Autodesk Fusion 360 part; units mm, degrees
note: some values were not read from the file. Set by a fixed rule: which sketch regions a step uses.
(part 15 of 15)
  line L12343 (-11.7716, -39.6941) -> (-12.0521, -39.6609)
  line L12344 (1.5382, -40.9023) -> (1.397, -40.7821)
  line L12345 (12.7412, -42.5744) -> (12.5951, -42.6886)
  line L12346 (11.5659, -41.0915) -> (11.7302, -41.0056)
  line L12347 (11.908, -40.9533) -> (12.0927, -40.9365)
  line L12348 (1.1512, -39.9247) -> (1.2072, -39.7479)
  line L12349 (1.397, -40.7821) -> (1.2819, -40.6368)
  line L12350 (11.2028, -42.2362) -> (11.1517, -42.0579)
  line L12351 (1.2072, -39.7479) -> (1.2966, -39.5855)
  line L12352 (1.2819, -40.6368) -> (1.1971, -40.4719)
  line L12353 (12.0662, -42.8362) -> (11.8821, -42.8143)
  line L12354 (2.424, -41.0079) -> (2.2454, -41.0578)
  line L12355 (1.5602, -39.3273) -> (1.7245, -39.2414)
  line L12356 (1.1971, -40.4719) -> (1.146, -40.2937)
  line L12357 (1.2966, -39.5855) -> (1.4157, -39.4434)
  line L12358 (-9.9098, -38.6322) -> (-10.0593, -38.8719)
  line L12359 (-9.7568, -37.1383) -> (-9.6973, -37.4145)
  line L12360 (-9.7956, -38.3738) -> (-9.9098, -38.6322)
  line L12361 (-12.8274, -39.3326) -> (-13.0464, -39.1543)
  line L12362 (1.146, -40.2937) -> (1.1305, -40.1089)
  line L12363 (-13.5251, -38.4617) -> (-13.6145, -38.1937)
  line L12364 (-13.6653, -37.9158) -> (-13.6764, -37.6335)
  line L12365 (1.7245, -39.2414) -> (1.9024, -39.189)
  line L12366 (11.7057, -42.757) -> (11.5439, -42.6665)
  line L12367 (-11.0893, -35.7847) -> (-10.8258, -35.8867)
  line L12368 (11.3022, -41.3497) -> (11.4214, -41.2077)
  line L12369 (11.8821, -42.8143) -> (11.7057, -42.757)
  line L12370 (1.8764, -41.05) -> (1.7001, -40.9927)
  line L12371 (2.7355, -40.8102) -> (2.5894, -40.9243)
  line L12372 (-11.3645, -35.7209) -> (-11.0893, -35.7847)
  line L12373 (2.9483, -40.5086) -> (2.8567, -40.6698)
  line L12374 (-10.8258, -35.8867) -> (-10.5793, -36.0247)
  line L12375 (1.7001, -40.9927) -> (1.5382, -40.9023)
  line L12376 (2.5894, -40.9243) -> (2.424, -41.0079)
  line L12377 (-10.1565, -36.3974) -> (-9.9887, -36.6247)
  line L12378 (3.0068, -40.3327) -> (2.9483, -40.5086)
  line L12379 (2.0605, -41.072) -> (1.8764, -41.05)
  line L12380 (-6.1433, -37.7909) -> (-6.0004, -37.9091)
  line L12381 (-16.025, -37.5022) -> (-16.1711, -37.6163)
  line L12382 (-9.6973, -37.4145) -> (-9.6774, -37.6963)
  line L12383 (-16.1711, -37.6163) -> (-16.3366, -37.6999)
  line L12384 (-7.6089, -38.7499) -> (-7.6244, -38.5652)
  line L12385 (-9.7189, -38.1019) -> (-9.7956, -38.3738)
  line L12386 (-7.4731, -39.0931) -> (-7.5578, -38.9282)
  line L12387 (-10.6864, -39.4336) -> (-10.9411, -39.5559)
  line L12388 (-5.7249, -38.605) -> (-5.7481, -38.7889)
  line L12389 (-5.8067, -38.9649) -> (-5.8982, -39.1261)
  line L12390 (-15.7538, -37.0247) -> (-15.8123, -37.2006)
  line L12391 (-7.4584, -38.0417) -> (-7.3392, -37.8997)
  line L12392 (-17.0605, -37.6847) -> (-17.2224, -37.5943)
  line L12393 (-17.2224, -37.5943) -> (-17.3635, -37.4741)
  line L12394 (-17.3635, -37.4741) -> (-17.4787, -37.3288)
  line L12395 (-17.4787, -37.3288) -> (-17.5635, -37.1639)
  line L12396 (-12.4716, -35.8608) -> (-12.2051, -35.7672)
  line L12397 (-10.4515, -39.2766) -> (-10.6864, -39.4336)
  line L12398 (-7.6038, -38.3809) -> (-7.5477, -38.2042)
  line L12399 (-13.4734, -36.8164) -> (-13.3315, -36.5722)
  line L12400 (-16.7001, -37.764) -> (-16.8842, -37.742)
  line L12401 (-9.6813, -37.8219) -> (-9.7189, -38.1019)
  line L12402 (-7.5477, -38.2042) -> (-7.4584, -38.0417)
  line L12403 (-5.7245, -38.5785) -> (-5.7249, -38.605)
  line L12404 (-17.5635, -37.1639) -> (-17.6146, -36.9857)
  line L12405 (-10.9411, -39.5559) -> (-11.2105, -39.6411)
  line L12406 (-13.0464, -39.1543) -> (-13.2382, -38.9468)
  line L12407 (-6.3064, -37.7027) -> (-6.1433, -37.7909)
  line L12408 (-5.7962, -38.2164) -> (-5.7426, -38.3939)
  line L12409 (-5.7426, -38.3939) -> (-5.7245, -38.5785)
  line L12410 (-7.3579, -39.2384) -> (-7.4731, -39.0931)
  line L12411 (-7.5578, -38.9282) -> (-7.6089, -38.7499)
  line L12412 (-15.8019, -36.4522) -> (-15.7483, -36.6297)
  line L12413 (-6.6679, -37.6285) -> (-6.4835, -37.6479)
  line L12414 (-15.8123, -37.2006) -> (-15.9039, -37.3618)
  line L12415 (-16.8842, -37.742) -> (-17.0605, -37.6847)
  line L12416 (-6.331, -39.4642) -> (-6.5096, -39.514)
  line L12417 (-5.8982, -39.1261) -> (-6.0194, -39.2664)
  line L12418 (-6.0004, -37.9091) -> (-5.8833, -38.0527)
  line L12419 (-11.928, -35.7121) -> (-11.6459, -35.6966)
  line L12420 (-6.6944, -39.5282) -> (-6.8785, -39.5063)
  line L12421 (-6.4835, -37.6479) -> (-6.3064, -37.7027)
  line L12422 (-11.6459, -35.6966) -> (-11.3645, -35.7209)
  line L12423 (-7.0549, -39.449) -> (-7.2167, -39.3585)
  line L12424 (-16.312, -35.9384) -> (-16.1489, -36.0266)
  line L12425 (-6.1655, -39.3806) -> (-6.331, -39.4642)
  line L12426 (-7.2167, -39.3585) -> (-7.3579, -39.2384)
  line L12427 (-11.4891, -39.6874) -> (-11.7716, -39.6941)
  line L12428 (-5.8833, -38.0527) -> (-5.7962, -38.2164)
  line L12429 (-6.5096, -39.514) -> (-6.6944, -39.5282)
  line L12430 (-12.9522, -36.1553) -> (-12.7223, -35.991)
  line L12431 (-12.2051, -35.7672) -> (-11.928, -35.7121)
  line L12432 (-16.5152, -37.7498) -> (-16.7001, -37.764)
  line L12433 (-12.7223, -35.991) -> (-12.4716, -35.8608)
  line L12434 (-16.1489, -36.0266) -> (-16.0061, -36.1448)
  line L12435 (-16.0061, -36.1448) -> (-15.8889, -36.2885)
  line L12436 (-15.9039, -37.3618) -> (-16.025, -37.5022)
  line L12437 (-15.7305, -36.8407) -> (-15.7538, -37.0247)
  line L12438 (-6.0194, -39.2664) -> (-6.1655, -39.3806)
  line L12439 (-13.6476, -37.3525) -> (-13.5795, -37.0783)
  line L12440 (-6.8785, -39.5063) -> (-7.0549, -39.449)
  line L12441 (-15.7483, -36.6297) -> (-15.7302, -36.8142)
  line L12442 (-5.7481, -38.7889) -> (-5.8067, -38.9649)
  line L12443 (-7.6244, -38.5652) -> (-7.6038, -38.3809)
  line L12444 (-17.464, -36.2775) -> (-17.3449, -36.1354)
  line L12445 (-16.3366, -37.6999) -> (-16.5152, -37.7498)
  line L12446 (-29.447, -36.1256) -> (-29.7017, -36.2479)
  line L12447 (-28.4379, -34.3883) -> (-28.4419, -34.5139)
  line L12448 (-30.4065, -32.3886) -> (-30.1251, -32.4129)
  line L12449 (-32.1594, -35.4064) -> (-32.2857, -35.1537)
  line L12450 (-24.9039, -34.4829) -> (-24.761, -34.6011)
  line L12451 (-31.2322, -32.5528) -> (-30.9657, -32.4592)
  line L12452 (-24.6438, -34.7447) -> (-24.5568, -34.9084)
  line L12453 (-31.0858, -36.2805) -> (-31.3459, -36.1703)
  line L12454 (-6.8525, -37.6453) -> (-6.6679, -37.6285)
  line L12455 (-31.7128, -32.8473) -> (-31.4829, -32.683)
  line L12456 (-25.2441, -34.3399) -> (-25.067, -34.3947)
  line L12457 (-24.5672, -35.6569) -> (-24.6588, -35.8181)
  line L12458 (-32.3401, -33.7703) -> (-32.234, -33.5084)
  line L12459 (-24.5087, -35.4809) -> (-24.5672, -35.6569)
  line L12460 (-31.9988, -35.6388) -> (-32.1594, -35.4064)
  line L12461 (-17.0361, -35.9334) -> (-16.8582, -35.881)
  line L12462 (-28.4579, -34.1065) -> (-28.4379, -34.3883)
  line L12463 (-28.7493, -33.3167) -> (-28.6151, -33.5653)
  line L12464 (-24.5568, -34.9084) -> (-24.5032, -35.0859)
  line L12465 (-32.234, -33.5084) -> (-32.0921, -33.2642)
  line L12466 (-24.4855, -35.297) -> (-24.5087, -35.4809)
  line L12467 (-31.807, -35.8463) -> (-31.9988, -35.6388)
  line L12468 (-29.7017, -36.2479) -> (-29.971, -36.3331)
  line L12469 (-29.2121, -35.9686) -> (-29.447, -36.1256)
  line L12470 (-29.971, -36.3331) -> (-30.2497, -36.3794)
  line L12471 (-32.4259, -34.6078) -> (-32.437, -34.3255)
  line L12472 (-28.9171, -33.0894) -> (-28.7493, -33.3167)
  line L12473 (-29.1153, -32.8881) -> (-28.9171, -33.0894)
  line L12474 (-28.5174, -33.8303) -> (-28.4579, -34.1065)
  line L12475 (-30.8127, -36.3529) -> (-31.0858, -36.2805)
  line L12476 (-7.3392, -37.8997) -> (-7.1947, -37.7835)
  line L12477 (-17.3449, -36.1354) -> (-17.2004, -36.0193)
  line L12478 (-30.5322, -36.3861) -> (-30.8127, -36.3529)
  line L12479 (-16.8582, -35.881) -> (-16.6735, -35.8642)
  line L12480 (-16.4892, -35.8836) -> (-16.312, -35.9384)
  line L12481 (-29.3399, -32.7167) -> (-29.1153, -32.8881)
  line L12482 (-30.2497, -36.3794) -> (-30.5322, -36.3861)
  line L12483 (-17.6301, -36.8009) -> (-17.6094, -36.6167)
  line L12484 (-28.4419, -34.5139) -> (-28.4795, -34.7939)
  line L12485 (-29.5864, -32.5787) -> (-29.3399, -32.7167)
  line L12486 (-15.7302, -36.8142) -> (-15.7305, -36.8407)
  line L12487 (-24.5032, -35.0859) -> (-24.4851, -35.2705)
  line L12488 (-31.3459, -36.1703) -> (-31.588, -36.0246)
  line L12489 (-15.8889, -36.2885) -> (-15.8019, -36.4522)
  line L12490 (-24.4851, -35.2705) -> (-24.4855, -35.297)
  line L12491 (-32.2857, -35.1537) -> (-32.3751, -34.8857)
  line L12492 (-28.6151, -33.5653) -> (-28.5174, -33.8303)
  line L12493 (-32.437, -34.3255) -> (-32.4082, -34.0445)
  line L12494 (-28.4795, -34.7939) -> (-28.5562, -35.0658)
  line L12495 (-17.5534, -36.4399) -> (-17.464, -36.2775)
  line L12496 (-30.1251, -32.4129) -> (-29.8499, -32.4767)
  line L12497 (-29.0017, -35.7802) -> (-29.2121, -35.9686)
  line L12498 (-16.6735, -35.8642) -> (-16.4892, -35.8836)
  line L12499 (-17.6094, -36.6167) -> (-17.5534, -36.4399)
  line L12500 (-17.2004, -36.0193) -> (-17.0361, -35.9334)
  line L12501 (-28.5562, -35.0658) -> (-28.6704, -35.3242)
  line L12502 (-28.6704, -35.3242) -> (-28.8199, -35.5639)
  line L12503 (-28.8199, -35.5639) -> (-29.0017, -35.7802)
  line L12504 (-29.8499, -32.4767) -> (-29.5864, -32.5787)
  line L12505 (-17.6146, -36.9857) -> (-17.6301, -36.8009)
  line L12506 (-7.1947, -37.7835) -> (-7.0304, -37.6976)
  line L12507 (-7.0304, -37.6976) -> (-6.8525, -37.6453)
  line L12508 (-26.3695, -35.442) -> (-26.385, -35.2572)
  line L12509 (-25.9553, -34.4755) -> (-25.791, -34.3896)
  line L12510 (-26.385, -35.2572) -> (-26.3644, -35.0729)
  line L12511 (-24.6588, -35.8181) -> (-24.78, -35.9584)
  line L12512 (-25.455, -36.2203) -> (-25.6391, -36.1983)
  line L12513 (-24.761, -34.6011) -> (-24.6438, -34.7447)
  line L12514 (-25.6391, -36.1983) -> (-25.8154, -36.141)
  line L12515 (-35.0726, -32.6304) -> (-34.9095, -32.7186)
  line L12516 (-36.2393, -34.0208) -> (-36.3241, -33.8559)
  line L12517 (-35.6448, -34.434) -> (-35.8211, -34.3767)
  line L12518 (-26.3083, -34.8962) -> (-26.219, -34.7337)
  line L12519 (-36.3241, -33.8559) -> (-36.3752, -33.6777)
  line L12520 (-36.1054, -32.8274) -> (-35.9609, -32.7113)
  line L12521 (-25.067, -34.3947) -> (-24.9039, -34.4829)
  line L12522 (-30.6886, -32.4041) -> (-30.4065, -32.3886)
  line L12523 (-48.347, -29.2707) -> (-48.1005, -29.4087)
  line L12524 (-47.6777, -29.7814) -> (-47.5099, -30.0087)
  line L12525 (-48.1005, -29.4087) -> (-47.8759, -29.5801)
  line L12526 (-34.5624, -33.1442) -> (-34.5089, -33.3217)
  line L12527 (-35.6188, -32.573) -> (-35.4341, -32.5562)
  line L12528 (-35.0972, -34.3919) -> (-35.2758, -34.4418)
  line L12529 (-47.5099, -30.0087) -> (-47.3757, -30.2573)
  line L12530 (-35.2758, -34.4418) -> (-35.4607, -34.456)
  line L12531 (-34.4908, -33.5062) -> (-34.4911, -33.5327)
  line L12532 (-31.9172, -33.0423) -> (-31.7128, -32.8473)
  line L12533 (-24.9261, -36.0726) -> (-25.0916, -36.1562)
  line L12534 (-25.4285, -34.3205) -> (-25.2441, -34.3399)
  line L12535 (-25.8154, -36.141) -> (-25.9773, -36.0506)
  line L12536 (-25.9773, -36.0506) -> (-26.1185, -35.9304)
  line L12537 (-26.3184, -35.6202) -> (-26.3695, -35.442)
  line L12538 (-34.9095, -32.7186) -> (-34.7667, -32.8368)
  line L12539 (-47.3757, -30.2573) -> (-47.2779, -30.5223)
  line L12540 (-34.7667, -32.8368) -> (-34.6495, -32.9805)
  line L12541 (-47.8759, -29.5801) -> (-47.6777, -29.7814)
  line L12542 (-35.7966, -32.6254) -> (-35.6188, -32.573)
  line L12543 (-34.6645, -34.0538) -> (-34.7856, -34.1942)
  line L12544 (-35.2497, -32.5756) -> (-35.0726, -32.6304)
  line L12545 (-31.588, -36.0246) -> (-31.807, -35.8463)
  line L12546 (-26.219, -34.7337) -> (-26.0998, -34.5917)
  line L12547 (-32.3751, -34.8857) -> (-32.4259, -34.6078)
  line L12548 (-34.6495, -32.9805) -> (-34.5624, -33.1442)
  line L12549 (-34.4911, -33.5327) -> (-34.5144, -33.7167)
  line L12550 (-26.1185, -35.9304) -> (-26.2337, -35.7851)
  line L12551 (-31.4829, -32.683) -> (-31.2322, -32.5528)
  line L12552 (-34.7856, -34.1942) -> (-34.9317, -34.3083)
  line L12553 (-25.2702, -36.206) -> (-25.455, -36.2203)
  line L12554 (-36.37, -33.3087) -> (-36.3139, -33.1319)
  line L12555 (-30.9657, -32.4592) -> (-30.6886, -32.4041)
  line L12556 (-26.2337, -35.7851) -> (-26.3184, -35.6202)
  line L12557 (-36.2246, -32.9695) -> (-36.1054, -32.8274)
  line L12558 (-25.0916, -36.1562) -> (-25.2702, -36.206)
  line L12559 (-25.791, -34.3896) -> (-25.6131, -34.3373)
  line L12560 (-32.0921, -33.2642) -> (-31.9172, -33.0423)
  line L12561 (-34.5089, -33.3217) -> (-34.4908, -33.5062)
  line L12562 (-34.9317, -34.3083) -> (-35.0972, -34.3919)
  line L12563 (-24.78, -35.9584) -> (-24.9261, -36.0726)
  line L12564 (-25.6131, -34.3373) -> (-25.4285, -34.3205)
  line L12565 (-47.2779, -30.5223) -> (-47.2185, -30.7985)
  line L12566 (-34.5729, -33.8926) -> (-34.6645, -34.0538)
  line L12567 (-35.4607, -34.456) -> (-35.6448, -34.434)
  line L12568 (-32.4082, -34.0445) -> (-32.3401, -33.7703)
  line L12569 (-26.0998, -34.5917) -> (-25.9553, -34.4755)
  line L12570 (-34.5144, -33.7167) -> (-34.5729, -33.8926)
  line L12571 (-26.3644, -35.0729) -> (-26.3083, -34.8962)
  line L12572 (-43.4194, -32.5101) -> (-43.5406, -32.6504)
  line L12573 (-43.5216, -31.2931) -> (-43.4044, -31.4367)
  line L12574 (-43.3278, -32.3489) -> (-43.4194, -32.5101)
  line L12575 (-35.9609, -32.7113) -> (-35.7966, -32.6254)
  line L12576 (-50.8527, -29.9562) -> (-50.6778, -29.7343)
  line L12577 (-50.4734, -29.5393) -> (-50.2435, -29.375)
  line L12578 (-49.8464, -32.9725) -> (-50.1065, -32.8623)
  line L12579 (-35.4341, -32.5562) -> (-35.2497, -32.5756)
  line L12580 (-45.1249, -31.7649) -> (-45.0689, -31.5882)
  line L12581 (-48.8857, -29.1049) -> (-48.6104, -29.1687)
  line L12582 (-43.2693, -32.1729) -> (-43.3278, -32.3489)
  line L12583 (-49.7263, -29.1512) -> (-49.4492, -29.0961)
  line L12584 (-43.6645, -31.1749) -> (-43.5216, -31.2931)
  line L12585 (-50.1065, -32.8623) -> (-50.3485, -32.7166)
  line L12586 (-36.3907, -33.4929) -> (-36.37, -33.3087)
  line L12587 (-47.9727, -32.6606) -> (-48.2076, -32.8176)
  line L12588 (-44.576, -32.833) -> (-44.7379, -32.7426)
  line L12589 (-49.4492, -29.0961) -> (-49.1671, -29.0806)
  line L12590 (-47.2025, -31.2059) -> (-47.2401, -31.4859)
  line L12591 (-47.3168, -31.7578) -> (-47.431, -32.0162)
  line L12592 (-36.3752, -33.6777) -> (-36.3907, -33.4929)
  line L12593 (-43.2461, -31.989) -> (-43.2693, -32.1729)
  line L12594 (-51.1357, -31.5777) -> (-51.1865, -31.2998)
  line L12595 (-44.8791, -32.6224) -> (-44.9942, -32.4771)
  line L12596 (-47.1985, -31.0803) -> (-47.2025, -31.2059)
  line L12597 (-50.2435, -29.375) -> (-49.9928, -29.2448)
  line L12598 (-47.431, -32.0162) -> (-47.5805, -32.2559)
  line L12599 (-49.2927, -33.0781) -> (-49.5733, -33.0449)
  line L12600 (-50.3485, -32.7166) -> (-50.5676, -32.5383)
  line L12601 (-51.1865, -31.2998) -> (-51.1975, -31.0175)
  line L12602 (-43.4044, -31.4367) -> (-43.3174, -31.6004)
  line L12603 (-48.2076, -32.8176) -> (-48.4623, -32.9399)
  line L12604 (-48.7316, -33.0251) -> (-49.0103, -33.0715)
  line L12605 (-45.1456, -31.9492) -> (-45.1249, -31.7649)
  line L12606 (-47.5805, -32.2559) -> (-47.7623, -32.4722)
  line L12607 (-48.6104, -29.1687) -> (-48.347, -29.2707)
  line L12608 (-48.4623, -32.9399) -> (-48.7316, -33.0251)
  line L12609 (-47.2185, -30.7985) -> (-47.1985, -31.0803)
  line L12610 (-44.3997, -32.8903) -> (-44.576, -32.833)
  line L12611 (-50.9946, -30.2004) -> (-50.8527, -29.9562)
  line L12612 (-50.5676, -32.5383) -> (-50.7594, -32.3308)
  line L12613 (-51.1975, -31.0175) -> (-51.1687, -30.7365)
  line L12614 (-44.0047, -31.0319) -> (-43.8276, -31.0867)
  line L12615 (-50.92, -32.0984) -> (-51.0463, -31.8457)
  line L12616 (-50.6778, -29.7343) -> (-50.4734, -29.5393)
  line L12617 (-43.2457, -31.9625) -> (-43.2461, -31.989)
  line L12618 (-51.0463, -31.8457) -> (-51.1357, -31.5777)
  line L12619 (-47.2401, -31.4859) -> (-47.3168, -31.7578)
  line L12620 (-44.9942, -32.4771) -> (-45.079, -32.3122)
  line L12621 (-36.1241, -34.1661) -> (-36.2393, -34.0208)
  line L12622 (-35.8211, -34.3767) -> (-35.9829, -34.2863)
  line L12623 (-43.8276, -31.0867) -> (-43.6645, -31.1749)
  line L12624 (-47.7623, -32.4722) -> (-47.9727, -32.6606)
  line L12625 (-51.1006, -30.4623) -> (-50.9946, -30.2004)
  line L12626 (-35.9829, -34.2863) -> (-36.1241, -34.1661)
  line L12627 (-51.1687, -30.7365) -> (-51.1006, -30.4623)
  line L12628 (-43.2638, -31.7779) -> (-43.2457, -31.9625)
  line L12629 (-45.079, -32.3122) -> (-45.1301, -32.134)
  line L12630 (-45.0689, -31.5882) -> (-44.9796, -31.4257)
  line L12631 (-45.1301, -32.134) -> (-45.1456, -31.9492)
  line L12632 (-50.7594, -32.3308) -> (-50.92, -32.0984)
  line L12633 (-36.3139, -33.1319) -> (-36.2246, -32.9695)
  line L12634 (-49.0103, -33.0715) -> (-49.2927, -33.0781)
  line L12635 (-49.5733, -33.0449) -> (-49.8464, -32.9725)
  line L12636 (-53.5462, -30.8862) -> (-53.6923, -31.0003)
  line L12637 (-53.4101, -29.6725) -> (-53.323, -29.8362)
  line L12638 (-54.0364, -31.1338) -> (-54.2212, -31.148)
  line L12639 (-54.5817, -31.0687) -> (-54.7435, -30.9783)
  line L12640 (-54.866, -29.5194) -> (-54.7215, -29.4033)
  line L12641 (-54.1947, -29.2482) -> (-54.0103, -29.2676)
  line L12642 (-53.6701, -29.4106) -> (-53.5273, -29.5288)
  line L12643 (-53.275, -30.4087) -> (-53.3335, -30.5846)
  line L12644 (-53.8578, -31.0839) -> (-54.0364, -31.1338)
  line L12645 (-54.9999, -30.7128) -> (-55.0846, -30.5479)
  line L12646 (-44.2156, -32.9123) -> (-44.3997, -32.8903)
  line L12647 (-54.7435, -30.9783) -> (-54.8847, -30.8581)
  line L12648 (-44.0307, -32.898) -> (-44.2156, -32.9123)
  line L12649 (-53.2514, -30.1982) -> (-53.2517, -30.2247)
  line L12650 (-49.9928, -29.2448) -> (-49.7263, -29.1512)
  line L12651 (-44.7379, -32.7426) -> (-44.8791, -32.6224)
  line L12652 (-43.8522, -32.8482) -> (-44.0307, -32.898)
  line L12653 (-44.9796, -31.4257) -> (-44.8604, -31.2837)
  line L12654 (-53.323, -29.8362) -> (-53.2694, -30.0137)
  line L12655 (-53.2517, -30.2247) -> (-53.275, -30.4087)
  line L12656 (-49.1671, -29.0806) -> (-48.8857, -29.1049)
  line L12657 (-55.0745, -29.8239) -> (-54.9852, -29.6615)
  line L12658 (-44.7159, -31.1675) -> (-44.5516, -31.0816)
  line L12659 (-53.6923, -31.0003) -> (-53.8578, -31.0839)
  line L12660 (-55.0846, -30.5479) -> (-55.1357, -30.3697)
  line L12661 (-53.3335, -30.5846) -> (-53.4251, -30.7458)
  line L12662 (-54.2212, -31.148) -> (-54.4053, -31.126)
  line L12663 (-54.9852, -29.6615) -> (-54.866, -29.5194)
  line L12664 (-54.0103, -29.2676) -> (-53.8332, -29.3224)
  line L12665 (-55.1306, -30.0007) -> (-55.0745, -29.8239)
  line L12666 (-54.7215, -29.4033) -> (-54.5572, -29.3174)
  line L12667 (-54.8847, -30.8581) -> (-54.9999, -30.7128)
  line L12668 (-55.1513, -30.1849) -> (-55.1306, -30.0007)
  line L12669 (-43.5406, -32.6504) -> (-43.6867, -32.7646)
  line L12670 (-44.3737, -31.0293) -> (-44.1891, -31.0125)
  line L12671 (-44.8604, -31.2837) -> (-44.7159, -31.1675)
  line L12672 (-43.6867, -32.7646) -> (-43.8522, -32.8482)
  line L12673 (-54.4053, -31.126) -> (-54.5817, -31.0687)
  line L12674 (-55.1357, -30.3697) -> (-55.1513, -30.1849)
  line L12675 (-44.5516, -31.0816) -> (-44.3737, -31.0293)
  line L12676 (-53.8332, -29.3224) -> (-53.6701, -29.4106)
  line L12677 (-53.5273, -29.5288) -> (-53.4101, -29.6725)
  line L12678 (-53.2694, -30.0137) -> (-53.2514, -30.1982)
  line L12679 (-53.4251, -30.7458) -> (-53.5462, -30.8862)
  line L12680 (-44.1891, -31.0125) -> (-44.0047, -31.0319)
  line L12681 (-54.3794, -29.265) -> (-54.1947, -29.2482)
  line L12682 (-54.5572, -29.3174) -> (-54.3794, -29.265)
  line L12683 (-43.3174, -31.6004) -> (-43.2638, -31.7779)
extrude "Extrude2" add sketch "atreuskeypad-F_Mask" along normal blind 6 contours L582 L583 L584 L585 L586 L587 L589 L591 L593 L595 L596 L598 L599 L600 L602 L603 L605 L606 L607 L609 L611 L612 L613 L617 L618 L621 L623 L624 L625 L626 L627 L629 L630 L631 L634 L643 L645 L651 L669 L672 L674 L679 L685 L687 L696 | L1022 L1035 L1036 L1037 L1038 L1040 L1041 L1042 L1043 L1044 L1045 L1046 L1047 L1048 L1049 L1050 L1051 L1052 L1053 L1054 L1055 L1056 L1057 L1058 L1059 L1060 L1061 L1062 L1063 L1064 L7754 L7784 L7923 L7925 L7928 L7933 L7934 L7935 L7937 L7939 L7945 L7946 L7948 L7949 L7951 | L2712 L2748 L2749 L2753 L2756 L2760 L2762 L2765 L2771 L2772 L2773 L2775 L2777 L2779 L2782 L2784 L2785 L2787 L2790 L2791 L2792 L2793 L2794 L2795 L2796 L2797 L2798 L2800 L2801 L2802 L2803 L2804 L2805 L2806 L2808 L2812 L2814 L2815 L2818 L2819 L2820 L2821 L2824 L2826 L2832 | L2770 L2774 L2776 L2778 L2780 L2781 L2783 L2786 L2788 L2789 L2799 L2807 L2809 L2810 L2811 L2813 L2816 L2817 L2822 L2823 L2825 L2827 L2828 L2829 L2830 L2831 L2833 L2835 L2836 L2837 L2838 L2839 L2840 L2841 L2842 L2845 L2847 L2849 L2850 L2851 L2852 L2855 L2860 L2865 L2867 | L3887 L3892 L3893 L3899 L3906 L3915 L3917 L3923 L3924 L3932 L3934 L3935 L3936 L3946 L3947 L3948 L3949 L3950 L3951 L3953 L3955 L3956 L3960 L3961 L3962 L3965 L3973 L3977 L3980 L3981 L3982 L3984 L3990 L3991 L3992 L3993 L3999 L4001 L4002 L4003 L4004 L4005 L4006 L4007 L4008 | L4192 L4195 L4197 L4198 L4200 L4201 L4206 L4207 L4211 L4212 L4214 L4229 L4240 L4241 L4249 L4250 L4254 L4256 L4257 L4258 L4260 L4261 L4262 L4263 L4264 L4266 L4270 L4271 L4278 L4279 L4284 L4285 L4286 L4288 L4293 L4294 L4295 L4296 L4297 L4302 L4305 L4307 L4308 L4311 L4312 | L4313 L4316 L4317 L4318 L4319 L4320 L4322 L4323 L4326 L4327 L4328 L4329 L4330 L4331 L4333 L4334 L4335 L4337 L4339 L4340 L4342 L4343 L4346 L4347 L4349 L4350 L4351 L4352 L4353 L4355 L4356 L4357 L4359 L4360 L4363 L4364 L4367 L4369 L4371 L4374 L4376 L4408 L4428 L4433 L4436 | L10536 L10537 L10538 L10539 L10540 L10541 L10542 L10543 L10544 L10545 L10546 L10550 L10551 L10552 L10554 L10555 L10556 L10557 L10559 L10560 L10562 L10566 L10567 L10568 L10569 L10570 L10573 L10574 L10576 L10577 L10579 L10580 L10582 L10583 L10584 L10585 L10586 L10589 L10590 L10593 L10596 L10597 L10599 L10637 L10651 | L10547 L10548 L10549 L10563 L10564 L10565 L10571 L10572 L10575 L10578 L10581 L10587 L10591 L10594 L10595 L10600 L10601 L10603 L10604 L10606 L10607 L10608 L10609 L10610 L10611 L10612 L10614 L10615 L10616 L10617 L10623 L10624 L10625 L10629 L10631 L10636 L10638 L10639 L10640 L10642 L10643 L10647 L10648 L10649 L10650 | L11932 L11937 L11939 L11940 L11941 L11944 L11945 L11947 L11948 L11952 L11953 L11954 L11957 L11959 L11965 L11967 L11973 L11976 L11979 L11981 L11983 L11991 L11992 L11996 L11999 L12005 L12006 L12014 L12015 L12016 L12017 L12019 L12020 L12024 L12027 L12028 L12031 L12032 L12036 L12039 L12042 L12045 L12046 L12057 L12058
sketch "Sketch4" plane through (0, 6, 0) normal (0, 1, 0) x (-1, 0, 0)
  line L0 (43.4815, 43.128) -> (43.6163, 43.3601)
  line L1 (43.6163, 43.3601) -> (43.717, 43.6089)
  line L2 (43.717, 43.6089) -> (43.7817, 43.8693)
  line L3 (43.7817, 43.8693) -> (43.8091, 44.1363)
  line L4 (43.8091, 44.1363) -> (43.7985, 44.4045)
  line L5 (43.7985, 44.4045) -> (43.7503, 44.6685)
  line L6 (43.7503, 44.6685) -> (43.6654, 44.9231)
  line L7 (43.6654, 44.9231) -> (43.5454, 45.1632)
  line L8 (43.5454, 45.1632) -> (43.3928, 45.384)
  line L9 (43.3928, 45.384) -> (43.2106, 45.581)
  line L10 (43.2106, 45.581) -> (43.0025, 45.7505)
  line L11 (43.0025, 45.7505) -> (42.7726, 45.8889)
  line L12 (42.7726, 45.8889) -> (42.5254, 45.9936)
  line L13 (42.5254, 45.9936) -> (42.266, 46.0623)
  line L14 (42.266, 46.0623) -> (41.9995, 46.0939)
  line L15 (41.9995, 46.0939) -> (41.7312, 46.0876)
  line L16 (41.7312, 46.0876) -> (41.4665, 46.0435)
  line L17 (41.4665, 46.0435) -> (41.2106, 45.9626)
  line L18 (41.2106, 45.9626) -> (40.9686, 45.8464)
  line L19 (40.9686, 45.8464) -> (40.7455, 45.6973)
  line L20 (40.7455, 45.6973) -> (40.5456, 45.5182)
  line L21 (40.5456, 45.5182) -> (40.3729, 45.3128)
  line L22 (40.3729, 45.3128) -> (40.2308, 45.0851)
  line L23 (40.2308, 45.0851) -> (40.1223, 44.8396)
  line L24 (40.1223, 44.8396) -> (40.0495, 44.5813)
  line L25 (40.0495, 44.5813) -> (40.0137, 44.3153)
  line L26 (40.0137, 44.3153) -> (40.01, 44.196)
  line L27 (40.01, 44.196) -> (40.029, 43.9283)
  line L28 (40.029, 43.9283) -> (40.0854, 43.6659)
  line L29 (40.0854, 43.6659) -> (40.1783, 43.4141)
  line L30 (40.1783, 43.4141) -> (40.3058, 43.1779)
  line L31 (40.3058, 43.1779) -> (40.4652, 42.962)
  line L32 (40.4652, 42.962) -> (40.6535, 42.7708)
  line L33 (40.6535, 42.7708) -> (40.8669, 42.608)
  line L34 (40.8669, 42.608) -> (41.101, 42.4768)
  line L35 (41.101, 42.4768) -> (41.3513, 42.38)
  line L36 (41.3513, 42.38) -> (41.6128, 42.3194)
  line L37 (41.6128, 42.3194) -> (41.8802, 42.2962)
  line L38 (41.8802, 42.2962) -> (42.1481, 42.311)
  line L39 (42.1481, 42.311) -> (42.4114, 42.3633)
  line L40 (42.4114, 42.3633) -> (42.6646, 42.4523)
  line L41 (42.6646, 42.4523) -> (42.9027, 42.576)
  line L42 (42.9027, 42.576) -> (43.1211, 42.732)
  line L43 (43.1211, 42.732) -> (43.3153, 42.9173)
  line L44 (43.3153, 42.9173) -> (43.4815, 43.128)
  circle A0 centre (41.9, 44.2) radius 3
  circle A1 centre (48.5, 82) radius 3
  circle A2 centre (-30.2, 113.3) radius 3
  circle A3 centre (-40.1, 56.9) radius 3
  circle A4 centre (-132.3, 151.1) radius 3
  circle A5 centre (-202.2, 150.8) radius 1.8358
  circle A6 centre (-202.2, 150.9) radius 3
  circle A7 centre (-307.3, 131.5) radius 2
  circle A8 centre (-307.3, 131.6) radius 3
  circle A9 centre (-294.1, 56.7) radius 3
  circle A10 centre (-153.6, 87.6) radius 2.0224
  circle A11 centre (-153.7, 87.6) radius 3
  circle A12 centre (-180.9, 87.3) radius 1.9105
  circle A13 centre (-180.8, 87.4) radius 3
  dimension "d5" = 6
  dimension "d6" = 6
  dimension "d7" = 6
  dimension "d8" = 6
  dimension "d9" = 6
  dimension "d10" = 6
  dimension "d11" = 6
  dimension "d12" = 6
  dimension "d13" = 6
  dimension "d14" = 6
  measures "d5" diameter of A0
  measures "d6" diameter of A1
  measures "d7" diameter of A2
  measures "d8" diameter of A3
  measures "d9" diameter of A4
  measures "d10" diameter of A6
  measures "d11" diameter of A8
  measures "d12" diameter of A9
  measures "d13" diameter of A11
  measures "d14" diameter of A13
extrude "Extrude3" add sketch "Sketch4" against normal blind 6 contours L0 L1 L2 L3 L4 L5 L6 L7 L8 L9 L10 L11 L12 L13 L14 L15 L16 L17 L18 L19 L20 L21 L22 L23 L24 L25 L26 L27 L28 L29 L30 L31 L32 L33 L34 L35 L36 L37 L38 L39 L40 L41 L42 L43 L44 | A0 | A1 | A2 | A3 | A4 | A5 | A6 | A7 | A8 | A9 | A10 | A11 | A12 | A13
sketch "Sketch5" plane through (0, 6, 0) normal (0, 1, 0) x (-1, 0, 0)
  circle A0 centre (41.9, 44.2) radius 3
  circle A1 centre (41.9, 44.2) radius 1.75
  circle A2 centre (48.5, 82) radius 1.75
  dimension "d17" = 3.5
  dimension "d18" = 3.5
  constraint concentric A0 A1
  measures "d17" diameter of A1
  measures "d18" diameter of A2
extrude "Extrude4" cut sketch "Sketch5" against normal blind 4 contours A1 | A2
sketch "Sketch6" plane through (0, 6, 0) normal (0, 1, 0) x (-1, 0, 0)
  circle A0 centre (-30.2, 113.3) radius 3
  circle A1 centre (-30.2, 113.3) radius 1.75
  dimension "d21" = 3.5
  constraint concentric A0 A1
  measures "d21" diameter of A1
extrude "Extrude5" cut sketch "Sketch6" against normal blind 4 contours A1
sketch "Sketch7" plane through (0, 6, 0) normal (0, 1, 0) x (-1, 0, 0)
  circle A0 centre (-40.1, 56.9) radius 3
  circle A1 centre (-40.1, 56.9) radius 1.75
  dimension "d24" = 3.5
  constraint concentric A0 A1
  measures "d24" diameter of A1
extrude "Extrude6" cut sketch "Sketch7" against normal blind 4 contours A1
sketch "Sketch8" plane through (0, 6, 0) normal (0, 1, 0) x (-1, 0, 0)
  circle A0 centre (-132.3, 151.1) radius 3
  circle A1 centre (-132.3, 151.1) radius 1.75
  dimension "d27" = 3.5
  constraint concentric A0 A1
  measures "d27" diameter of A1
extrude "Extrude7" cut sketch "Sketch8" against normal blind 4 contours A1
sketch "Sketch9" plane through (0, 6, 0) normal (0, 1, 0) x (-1, 0, 0)
  circle A0 centre (-153.7, 87.6) radius 3
  circle A1 centre (-153.7, 87.6) radius 1.75
  dimension "d30" = 3.5
  constraint concentric A0 A1
  measures "d30" diameter of A1
extrude "Extrude8" cut sketch "Sketch9" against normal blind 4 contours A1
sketch "Sketch10" plane through (0, 6, 0) normal (0, 1, 0) x (-1, 0, 0)
  circle A0 centre (-180.8, 87.4) radius 3
  circle A1 centre (-180.8, 87.4) radius 1.75
  dimension "d33" = 3.5
  constraint concentric A0 A1
  measures "d33" diameter of A1
extrude "Extrude9" cut sketch "Sketch10" against normal blind 4 contours A1
sketch "Sketch11" plane through (0, 6, 0) normal (0, 1, 0) x (-1, 0, 0)
  circle A0 centre (-202.2, 150.9) radius 3
  circle A1 centre (-202.2, 150.9) radius 1.75
  dimension "d36" = 3.5
  constraint concentric A0 A1
  measures "d36" diameter of A1
extrude "Extrude10" cut sketch "Sketch11" against normal blind 4 contours A1
sketch "Sketch12" plane through (0, 6, 0) normal (0, 1, 0) x (-1, 0, 0)
  circle A0 centre (-294.1, 56.7) radius 3
  circle A1 centre (-294.1, 56.7) radius 1.75
  dimension "d39" = 3.5
  constraint concentric A0 A1
  measures "d39" diameter of A1
extrude "Extrude11" cut sketch "Sketch12" against normal blind 4 contours A1
sketch "Sketch13" plane through (0, 6, 0) normal (0, 1, 0) x (-1, 0, 0)
  circle A0 centre (-307.3, 131.6) radius 3
  circle A1 centre (-307.3, 131.6) radius 1.75
  dimension "d42" = 3.5
  constraint concentric A0 A1
  measures "d42" diameter of A1
extrude "Extrude12" cut sketch "Sketch13" against normal blind 4 contours A1
sketch "Sketch14" plane through (0, 3, 0) normal (0, 1, 0) x (-1, 0, 0)
  circle A0 centre (-294.1, 56.7) radius 3
  circle A1 centre (-202.2, 150.9) radius 3
  circle A2 centre (48.5, 82) radius 3
  circle A3 centre (-30.2, 113.3) radius 3
  circle A4 centre (-307.3, 131.6) radius 3
  circle A5 centre (-153.7, 87.6) radius 3
  circle A6 centre (-132.3, 151.1) radius 3
  circle A7 centre (41.9, 44.2) radius 3
  circle A8 centre (-40.1, 56.9) radius 3
  circle A9 centre (-180.8, 87.4) radius 3
  line L0 (-252.037, 37.2596) -> (-233.271, 40.5889)
  line L1 (-233.271, 40.5889) -> (-177.793, 54.9784)
  line L2 (-177.793, 54.9784) -> (-177.784, 54.9772)
  line L3 (-177.784, 54.9772) -> (-177.776, 54.9799)
  line L4 (-177.776, 54.9799) -> (-177.766, 54.9747)
  line L5 (-177.766, 54.9747) -> (-177.755, 54.9731)
  line L6 (-177.755, 54.9731) -> (-177.75, 54.9664)
  line L7 (-177.75, 54.9664) -> (-177.742, 54.9626)
  line L8 (-177.742, 54.9626) -> (-176.107, 53.06)
  line L9 (-176.107, 53.06) -> (-158.184, 53.07)
  line L10 (-158.184, 53.07) -> (-156.659, 54.9317)
  line L11 (-156.659, 54.9317) -> (-156.651, 54.9359)
  line L12 (-156.651, 54.9359) -> (-156.645, 54.9431)
  line L13 (-156.645, 54.9431) -> (-156.635, 54.9446)
  line L14 (-156.635, 54.9446) -> (-156.625, 54.9498)
  line L15 (-156.625, 54.9498) -> (-156.616, 54.9471)
  line L16 (-156.616, 54.9471) -> (-156.607, 54.9484)
  line L17 (-156.607, 54.9484) -> (-101.099, 40.5089)
  line L18 (-101.099, 40.5089) -> (-82.3243, 37.2098)
  line L19 (-82.3243, 37.2098) -> (-63.1672, 36.1399)
  line L20 (-63.1672, 36.1399) -> (-63.1661, 36.1394)
  line L21 (-63.1661, 36.1394) -> (-63.165, 36.1397)
  line L22 (-63.165, 36.1397) -> (-25.155, 32.2997)
  line L23 (-25.155, 32.2997) -> (-25.1539, 32.2991)
  line L24 (-25.1539, 32.2991) -> (-25.1526, 32.2995)
  line L25 (-25.1526, 32.2995) -> (56.8492, 20.0866)
  line L26 (56.8492, 20.0866) -> (73.4021, 113.779)
  line L27 (73.4021, 113.779) -> (-1.5787, 127.041)
  line L28 (-1.5787, 127.041) -> (-1.5873, 127.046)
  line L29 (-1.5873, 127.046) -> (-1.5973, 127.048)
  line L30 (-1.5973, 127.048) -> (-1.6028, 127.056)
  line L31 (-1.6028, 127.056) -> (-1.611, 127.061)
  line L32 (-1.611, 127.061) -> (-1.6132, 127.071)
  line L33 (-1.6132, 127.071) -> (-1.6189, 127.08)
  line L34 (-1.6189, 127.08) -> (-5.3719, 144.767)
  line L35 (-5.3719, 144.767) -> (-42.8483, 151.381)
  line L36 (-42.8483, 151.381) -> (-80.508, 157.491)
  line L37 (-80.508, 157.491) -> (-80.5123, 157.493)
  line L38 (-80.5123, 157.493) -> (-80.5173, 157.493)
  line L39 (-80.5173, 157.493) -> (-142.939, 180.48)
  line L40 (-142.939, 180.48) -> (-191.71, 180.73)
  line L41 (-191.71, 180.73) -> (-253.501, 155.304)
  line L42 (-253.501, 155.304) -> (-253.508, 155.304)
  line L43 (-253.508, 155.304) -> (-253.515, 155.3)
  line L44 (-253.515, 155.3) -> (-291.513, 151.41)
  line L45 (-291.513, 151.41) -> (-328.992, 144.819)
  line L46 (-328.992, 144.819) -> (-309.159, 32.3537)
  line L47 (-309.159, 32.3537) -> (-252.037, 37.2596)
  line L48 (-25.5891, 27.9801) -> (-24.8439, 28.2094)
  line L49 (-24.8439, 28.2094) -> (60.1108, 15.5567)
  line L50 (60.1108, 15.5567) -> (78.0369, 117.0213)
  line L51 (78.0369, 117.0213) -> (1.7411, 130.5159)
  line L52 (1.7411, 130.5159) -> (-2.0192, 148.2371)
  line L53 (-2.0192, 148.2371) -> (-42.1804, 155.3249)
  line L54 (-42.1804, 155.3249) -> (-79.322, 161.3509)
  line L55 (-79.322, 161.3509) -> (-79.6276, 161.493)
  line L56 (-79.6276, 161.493) -> (-79.8042, 161.493)
  line L57 (-79.8042, 161.493) -> (-142.216, 184.4763)
  line L58 (-142.216, 184.4763) -> (-192.4909, 184.7341)
  line L59 (-192.4909, 184.7341) -> (-254.2918, 159.304)
  line L60 (-254.2918, 159.304) -> (-254.5703, 159.304)
  line L61 (-254.5703, 159.304) -> (-254.7645, 159.193)
  line L62 (-254.7645, 159.193) -> (-292.0638, 155.3745)
  line L63 (-292.0638, 155.3745) -> (-333.6262, 148.0654)
  line L64 (-333.6262, 148.0654) -> (-312.4627, 28.0552)
  line L65 (-312.4627, 28.0552) -> (-251.5154, 33.2897)
  line L66 (-251.5154, 33.2897) -> (-232.4182, 36.6777)
  line L67 (-232.4182, 36.6777) -> (-179.1713, 50.4886)
  line L68 (-179.1713, 50.4886) -> (-177.9428, 49.059)
  line L69 (-177.9428, 49.059) -> (-156.289, 49.0711)
  line L70 (-156.289, 49.0711) -> (-155.1671, 50.4407)
  line L71 (-155.1671, 50.4407) -> (-101.95, 36.5972)
  line L72 (-101.95, 36.5972) -> (-82.7836, 33.2292)
  line L73 (-82.7836, 33.2292) -> (-64.1394, 32.188)
  line L74 (-64.1394, 32.188) -> (-63.5067, 31.9004)
  line L75 (-63.5067, 31.9004) -> (-62.8286, 32.0854)
  line L76 (-62.8286, 32.0854) -> (-26.361, 28.4012)
  line L77 (-26.361, 28.4012) -> (-25.5891, 27.9801)
  dimension "d45" = 4
extrude "Extrude13" add sketch "Sketch14" against normal blind 3 contours L48 L49 L50 L51 L52 L53 L54 L55 L56 L57 L58 L59 L60 L61 L62 L63 L64 L65 L66 L67 L68 L69 L70 L71 L72 L73 L74 L75 L76 L77
sketch "Sketch15" plane through (0, 3, 0) normal (0, 1, 0) x (-1, 0, 0)
  line L0 (-26.361, 28.4012) -> (-25.5891, 27.9801)
  line L1 (-25.5891, 27.9801) -> (-24.8439, 28.2094)
  line L2 (-24.8439, 28.2094) -> (60.1108, 15.5567)
  line L3 (60.1108, 15.5567) -> (78.0369, 117.0213)
  line L4 (78.0369, 117.0213) -> (1.7411, 130.5159)
  line L5 (1.7411, 130.5159) -> (-2.0192, 148.2371)
  line L6 (-2.0192, 148.2371) -> (-42.1804, 155.3249)
  line L7 (-42.1804, 155.3249) -> (-79.322, 161.3509)
  line L8 (-79.322, 161.3509) -> (-79.6276, 161.493)
  line L9 (-79.6276, 161.493) -> (-79.8042, 161.493)
  line L10 (-79.8042, 161.493) -> (-142.216, 184.4763)
  line L11 (-142.216, 184.4763) -> (-192.4909, 184.7341)
  line L12 (-192.4909, 184.7341) -> (-254.2918, 159.304)
  line L13 (-254.2918, 159.304) -> (-254.5703, 159.304)
  line L14 (-254.5703, 159.304) -> (-254.7645, 159.193)
  line L15 (-254.7645, 159.193) -> (-292.0638, 155.3745)
  line L16 (-292.0638, 155.3745) -> (-333.6262, 148.0654)
  line L17 (-333.6262, 148.0654) -> (-312.4627, 28.0552)
  line L18 (-312.4627, 28.0552) -> (-251.5154, 33.2897)
  line L19 (-251.5154, 33.2897) -> (-232.4182, 36.6777)
  line L20 (-232.4182, 36.6777) -> (-179.1713, 50.4886)
  line L21 (-179.1713, 50.4886) -> (-177.9428, 49.059)
  line L22 (-177.9428, 49.059) -> (-156.289, 49.0711)
  line L23 (-156.289, 49.0711) -> (-155.1671, 50.4407)
  line L24 (-155.1671, 50.4407) -> (-101.95, 36.5972)
  line L25 (-101.95, 36.5972) -> (-82.7836, 33.2292)
  line L26 (-82.7836, 33.2292) -> (-64.1394, 32.188)
  line L27 (-64.1394, 32.188) -> (-63.5067, 31.9004)
  line L28 (-63.5067, 31.9004) -> (-62.8286, 32.0854)
  line L29 (-62.8286, 32.0854) -> (-26.361, 28.4012)
  circle A0 centre (-294.1, 56.7) radius 3
  circle A1 centre (-202.2, 150.9) radius 3
  circle A2 centre (48.5, 82) radius 3
  circle A3 centre (-30.2, 113.3) radius 3
  circle A4 centre (-307.3, 131.6) radius 3
  circle A5 centre (-153.7, 87.6) radius 3
  circle A6 centre (-132.3, 151.1) radius 3
  circle A7 centre (41.9, 44.2) radius 3
  circle A8 centre (-40.1, 56.9) radius 3
  circle A9 centre (-180.8, 87.4) radius 3
  line L30 (75.7195, 115.4002) -> (0.0646, 128.7814)
  line L31 (0.0646, 128.7814) -> (-3.6955, 146.5021)
  line L32 (-3.6955, 146.5021) -> (-42.5143, 153.353)
  line L33 (-42.5143, 153.353) -> (-79.915, 159.4209)
  line L34 (-79.915, 159.4209) -> (-80.0699, 159.493)
  line L35 (-80.0699, 159.493) -> (-80.1608, 159.493)
  line L36 (-80.1608, 159.493) -> (-142.5775, 182.4782)
  line L37 (-142.5775, 182.4782) -> (-192.1005, 182.732)
  line L38 (-192.1005, 182.732) -> (-253.8964, 157.304)
  line L39 (-253.8964, 157.304) -> (-254.0391, 157.304)
  line L40 (-254.0391, 157.304) -> (-254.1398, 157.2465)
  line L41 (-254.1398, 157.2465) -> (-291.7884, 153.3923)
  line L42 (-291.7884, 153.3923) -> (-331.3091, 146.4422)
  line L43 (-331.3091, 146.4422) -> (-310.8108, 30.2045)
  line L44 (-310.8108, 30.2045) -> (-251.7762, 35.2746)
  line L45 (-251.7762, 35.2746) -> (-232.8446, 38.6333)
  line L46 (-232.8446, 38.6333) -> (-178.4668, 52.7374)
  line L47 (-178.4668, 52.7374) -> (-177.0249, 51.0595)
  line L48 (-177.0249, 51.0595) -> (-157.2365, 51.0705)
  line L49 (-157.2365, 51.0705) -> (-155.9028, 52.6987)
  line L50 (-155.9028, 52.6987) -> (-101.5245, 38.553)
  line L51 (-101.5245, 38.553) -> (-82.5539, 35.2195)
  line L52 (-82.5539, 35.2195) -> (-63.6533, 34.1639)
  line L53 (-63.6533, 34.1639) -> (-63.3364, 34.0199)
  line L54 (-63.3364, 34.0199) -> (-62.9968, 34.1125)
  line L55 (-62.9968, 34.1125) -> (-25.758, 30.3504)
  line L56 (-25.758, 30.3504) -> (-25.3715, 30.1396)
  line L57 (-25.3715, 30.1396) -> (-24.9983, 30.2545)
  line L58 (-24.9983, 30.2545) -> (58.48, 17.8217)
  line L59 (58.48, 17.8217) -> (75.7195, 115.4002)
  dimension "d48" = -2
extrude "Extrude14" add sketch "Sketch15" along normal blind 6 contours L0 L1 L2 L3 L4 L5 L6 L7 L8 L9 L10 L11 L12 L13 L14 L15 L16 L17 L18 L19 L20 L21 L22 L23 L24 L25 L26 L27 L28 L29
sketch "Sketch16" plane through (0, 9, 0) normal (0, 1, 0) x (-1, 0, 0)
  line L0 (75.7195, 115.4002) -> (58.48, 17.8217)
  line L1 (58.48, 17.8217) -> (-24.9983, 30.2545)
  line L2 (-24.9983, 30.2545) -> (-25.3715, 30.1396)
  line L3 (-25.3715, 30.1396) -> (-25.758, 30.3504)
  line L4 (-25.758, 30.3504) -> (-62.9968, 34.1125)
  line L5 (-62.9968, 34.1125) -> (-63.3364, 34.0199)
  line L6 (-63.3364, 34.0199) -> (-63.6533, 34.1639)
  line L7 (-63.6533, 34.1639) -> (-82.5539, 35.2195)
  line L8 (-82.5539, 35.2195) -> (-101.5245, 38.553)
  line L9 (-101.5245, 38.553) -> (-155.9028, 52.6987)
  line L10 (-155.9028, 52.6987) -> (-157.2365, 51.0705)
  line L11 (-157.2365, 51.0705) -> (-177.0249, 51.0595)
  line L12 (-177.0249, 51.0595) -> (-178.4668, 52.7374)
  line L13 (-178.4668, 52.7374) -> (-232.8446, 38.6333)
  line L14 (-232.8446, 38.6333) -> (-251.7762, 35.2746)
  line L15 (-251.7762, 35.2746) -> (-310.8108, 30.2045)
  line L16 (-310.8108, 30.2045) -> (-331.3091, 146.4422)
  line L17 (-331.3091, 146.4422) -> (-291.7884, 153.3923)
  line L18 (-291.7884, 153.3923) -> (-254.1398, 157.2465)
  line L19 (-254.1398, 157.2465) -> (-254.0391, 157.304)
  line L20 (-254.0391, 157.304) -> (-253.8964, 157.304)
  line L21 (-253.8964, 157.304) -> (-192.1005, 182.732)
  line L22 (-192.1005, 182.732) -> (-142.5775, 182.4782)
  line L23 (-142.5775, 182.4782) -> (-80.1608, 159.493)
  line L24 (-80.1608, 159.493) -> (-80.0699, 159.493)
  line L25 (-80.0699, 159.493) -> (-79.915, 159.4209)
  line L26 (-79.915, 159.4209) -> (-42.5143, 153.353)
  line L27 (-42.5143, 153.353) -> (-3.6955, 146.5021)
  line L28 (-3.6955, 146.5021) -> (0.0646, 128.7814)
  line L29 (0.0646, 128.7814) -> (75.7195, 115.4002)
  line L30 (-62.8286, 32.0854) -> (-26.361, 28.4012)
  line L31 (-26.361, 28.4012) -> (-25.5891, 27.9801)
  line L32 (-25.5891, 27.9801) -> (-24.8439, 28.2094)
  line L33 (-24.8439, 28.2094) -> (60.1108, 15.5567)
  line L34 (60.1108, 15.5567) -> (78.0369, 117.0213)
  line L35 (78.0369, 117.0213) -> (1.7411, 130.5159)
  line L36 (1.7411, 130.5159) -> (-2.0192, 148.2371)
  line L37 (-2.0192, 148.2371) -> (-42.1804, 155.3249)
  line L38 (-42.1804, 155.3249) -> (-79.322, 161.3509)
  line L39 (-79.322, 161.3509) -> (-79.6276, 161.493)
  line L40 (-79.6276, 161.493) -> (-79.8042, 161.493)
  line L41 (-79.8042, 161.493) -> (-142.216, 184.4763)
  line L42 (-142.216, 184.4763) -> (-192.4909, 184.7341)
  line L43 (-192.4909, 184.7341) -> (-254.2918, 159.304)
  line L44 (-254.2918, 159.304) -> (-254.5703, 159.304)
  line L45 (-254.5703, 159.304) -> (-254.7645, 159.193)
  line L46 (-254.7645, 159.193) -> (-292.0638, 155.3745)
  line L47 (-292.0638, 155.3745) -> (-333.6262, 148.0654)
  line L48 (-333.6262, 148.0654) -> (-312.4627, 28.0552)
  line L49 (-312.4627, 28.0552) -> (-251.5154, 33.2897)
  line L50 (-251.5154, 33.2897) -> (-232.4182, 36.6777)
  line L51 (-232.4182, 36.6777) -> (-179.1713, 50.4886)
  line L52 (-179.1713, 50.4886) -> (-177.9428, 49.059)
  line L53 (-177.9428, 49.059) -> (-156.289, 49.0711)
  line L54 (-156.289, 49.0711) -> (-155.1671, 50.4407)
  line L55 (-155.1671, 50.4407) -> (-101.95, 36.5972)
  line L56 (-101.95, 36.5972) -> (-82.7836, 33.2292)
  line L57 (-82.7836, 33.2292) -> (-64.1394, 32.188)
  line L58 (-64.1394, 32.188) -> (-63.5067, 31.9004)
  line L59 (-63.5067, 31.9004) -> (-62.8286, 32.0854)
  line L60 (-158.5, 48.5) -> (-175.9766, 48.4902)
  line L61 (-175.9766, 48.4902) -> (-175.9785, 51.866)
  line L62 (-175.9785, 51.866) -> (-158.5, 51.8758)
  line L63 (-158.5, 51.8758) -> (-158.5, 48.5)
  constraint parallel L53 L60
  constraint perpendicular L11 L61
  constraint perpendicular L61 L62
  constraint vertical L63
extrude "Extrude15" cut sketch "Sketch16" against normal blind 4 contours L11 L53 L61 L63 | L11 L61 L62 L63 | L53 L60 L61 L63
extrude "Extrude16" add 1 faces at (164.326, 5, 50.3999) along direction (0, 1, 0) blind 1
